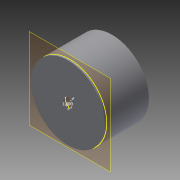
# Autodesk Inventor part: reel bs made by vecch
Saved by Autodesk Inventor 2015 (Build 190159000, 159)
## iProperties
Created: 2015-01-24
Part Number: reel bs made by vecch
Material: Generic
Document SubType Name: Modeling
Designer: Guest
Density: 1 g/cm^3
Appearance: Default
Author: Guest
Autodesk Inventor part; units mm, degrees
ref_plane "YZ Plane" through (0, 0, 0) normal (1, 0, 0) x (0, 1, 0)
ref_plane "XZ Plane" through (0, 0, 0) normal (0, 1, 0) x (-1, 0, 0)
ref_plane "XY Plane" through (0, 0, 0) normal (0, 0, 1) x (1, 0, 0)
ref_plane "Work Plane1" through (0, 0, 0) normal (0, 0, 1) x (1, 0, 0)
sketch "Sketch1" plane through (0, 0, 0) normal (0, 0, 1) x (1, 0, 0)
  line L0 (-2.3812, -10.3188) -> (-2.3813, -7.6374) projected
  arc A0 (2.3813, -7.6374) -> (-2.3813, -7.6374) centre (0, 0) ccw projected
  line L1 (2.3813, -7.6374) -> (2.3813, -10.3188) projected
  line L2 (2.3813, -10.3188) -> (-2.3812, -10.3188) projected
  circle A1 centre (0, 0) radius 12.7003 projected
  circle A2 centre (0, 0) radius 63.5
  dimension "d0" = 127
  constraints: 1 centre point, 1 coincident
  measures "d0" diameter of A2
extrude "Extrusion1" add sketch "Sketch1" along normal blind 76.2 contours A1 | A2
ref_plane "Work Plane2" through (0, 0, 73.025) normal (0, 0, 1) x (1, 0, 0)
sketch "Sketch2" plane through (0, 0, 73.025) normal (0, 0, 1) x (1, 0, 0)
  arc A0 (2.3813, -7.6374) -> (-2.3813, -7.6374) centre (0, 0) ccw projected
  circle A1 centre (0, 0) radius 12.7
  arc A2 (2.3813, -7.6374) -> (-2.3813, -7.6374) centre (0, 0) ccw projected
  line L0 (2.3813, -7.6374) -> (2.3813, -10.3188) projected
  line L1 (2.3813, -10.3188) -> (-2.3813, -10.3188) projected
  line L2 (-2.3813, -10.3188) -> (-2.3813, -7.6374) projected
  circle A3 centre (0, 0) radius 63.5 projected
  dimension "d4" = 25.4
  constraints: 1 centre point, 1 coincident
  measures "d4" diameter of A1
extrude "Extrusion2" cut sketch "Sketch2" against normal blind 69.85 contours A3
body "Solid1"
